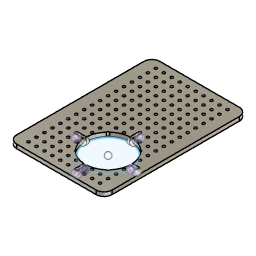
base-plate-2 (Autodesk Fusion 360 design; units mm, degrees)
part number: 2026-04-18-13-53-20-115
Autodesk Fusion 360 part; units mm, degrees
sketch "Sketch1" plane through (0, 0, 0) normal (0, 0, 1) x (1, 0, 0)
  line L0 (10, 0) -> (110, 0)
  line L1 (120, 10) -> (120, 170)
  line L2 (110, 180) -> (10, 180)
  line L3 (0, 170) -> (0, 10)
  arc A0 (10, 180) -> (0, 170) centre (10, 170) ccw
  arc A1 (120, 170) -> (110, 180) centre (110, 170) ccw
  arc A2 (110, 0) -> (120, 10) centre (110, 10) ccw
  arc A3 (0, 10) -> (10, 0) centre (10, 10) ccw
  circle A4 centre (15, 170) radius 1.625
  circle A5 centre (25, 170) radius 1.625
  circle A6 centre (35, 170) radius 1.625
  circle A7 centre (45, 170) radius 1.625
  circle A8 centre (65, 170) radius 1.625
  circle A9 centre (55, 170) radius 1.625
  circle A10 centre (35, 100) radius 1.625
  circle A11 centre (25, 100) radius 1.625
  circle A12 centre (15, 100) radius 1.625
  circle A13 centre (55, 100) radius 1.625
  circle A14 centre (65, 100) radius 1.625
  circle A15 centre (45, 100) radius 1.625
  circle A16 centre (15, 90) radius 1.625
  circle A17 centre (65, 90) radius 1.625
  circle A18 centre (65, 80) radius 1.625
  circle A19 centre (25, 90) radius 1.625
  circle A20 centre (45, 80) radius 1.625
  circle A21 centre (15, 80) radius 1.625
  circle A22 centre (35, 80) radius 1.625
  circle A23 centre (35, 90) radius 1.625
  circle A24 centre (55, 80) radius 1.625
  circle A25 centre (45, 90) radius 1.625
  circle A26 centre (25, 80) radius 1.625
  circle A27 centre (55, 90) radius 1.625
  circle A28 centre (35, 50) radius 1.625
  circle A29 centre (15, 50) radius 1.625
  circle A30 centre (65, 40) radius 1.625
  circle A31 centre (35, 40) radius 1.625
  circle A32 centre (25, 60) radius 1.625
  circle A33 centre (25, 50) radius 1.625
  circle A34 centre (45, 40) radius 1.625
  circle A35 centre (45, 60) radius 1.625
  circle A36 centre (15, 40) radius 1.625
  circle A37 centre (65, 50) radius 1.625
  circle A38 centre (25, 40) radius 1.625
  circle A39 centre (55, 50) radius 1.625
  circle A40 centre (45, 50) radius 1.625
  circle A41 centre (55, 40) radius 1.625
  circle A42 centre (15, 70) radius 1.625
  circle A43 centre (45, 70) radius 1.625
  circle A44 centre (65, 60) radius 1.625
  circle A45 centre (25, 70) radius 1.625
  circle A46 centre (55, 70) radius 1.625
  circle A47 centre (65, 70) radius 1.625
  circle A48 centre (15, 60) radius 1.625
  circle A49 centre (55, 60) radius 1.625
  circle A50 centre (35, 60) radius 1.625
  circle A51 centre (35, 70) radius 1.625
  circle A52 centre (25, 10) radius 1.625
  circle A53 centre (55, 20) radius 1.625
  circle A54 centre (25, 20) radius 1.625
  circle A55 centre (35, 20) radius 1.625
  circle A56 centre (35, 30) radius 1.625
  circle A57 centre (55, 30) radius 1.625
  circle A58 centre (55, 10) radius 1.625
  circle A59 centre (15, 30) radius 1.625
  circle A60 centre (65, 30) radius 1.625
  circle A61 centre (45, 10) radius 1.625
  circle A62 centre (15, 10) radius 1.625
  circle A63 centre (45, 20) radius 1.625
  circle A64 centre (45, 30) radius 1.625
  circle A65 centre (15, 20) radius 1.625
  circle A66 centre (65, 10) radius 1.625
  circle A67 centre (65, 20) radius 1.625
  circle A68 centre (35, 10) radius 1.625
  circle A69 centre (25, 30) radius 1.625
  circle A70 centre (35, 110) radius 1.625
  circle A71 centre (65, 110) radius 1.625
  circle A72 centre (15, 120) radius 1.625
  circle A73 centre (65, 120) radius 1.625
  circle A74 centre (45, 120) radius 1.625
  circle A75 centre (25, 130) radius 1.625
  circle A76 centre (55, 130) radius 1.625
  circle A77 centre (25, 110) radius 1.625
  circle A78 centre (65, 140) radius 1.625
  circle A79 centre (25, 120) radius 1.625
  circle A80 centre (35, 140) radius 1.625
  circle A81 centre (15, 140) radius 1.625
  circle A82 centre (15, 130) radius 1.625
  circle A83 centre (25, 140) radius 1.625
  circle A84 centre (45, 130) radius 1.625
  circle A85 centre (55, 140) radius 1.625
  circle A86 centre (55, 110) radius 1.625
  circle A87 centre (65, 130) radius 1.625
  circle A88 centre (45, 140) radius 1.625
  circle A89 centre (45, 110) radius 1.625
  circle A90 centre (35, 120) radius 1.625
  circle A91 centre (15, 110) radius 1.625
  circle A92 centre (55, 120) radius 1.625
  circle A93 centre (35, 130) radius 1.625
  circle A94 centre (45, 150) radius 1.625
  circle A95 centre (65, 140) radius 1.625
  circle A96 centre (55, 140) radius 1.625
  circle A97 centre (65, 150) radius 1.625
  circle A98 centre (45, 140) radius 1.625
  circle A99 centre (55, 150) radius 1.625
  circle A100 centre (55, 160) radius 1.625
  circle A101 centre (35, 140) radius 1.625
  circle A102 centre (35, 150) radius 1.625
  circle A103 centre (35, 160) radius 1.625
  circle A104 centre (15, 140) radius 1.625
  circle A105 centre (25, 140) radius 1.625
  circle A106 centre (45, 160) radius 1.625
  circle A107 centre (15, 160) radius 1.625
  circle A108 centre (15, 150) radius 1.625
  circle A109 centre (25, 150) radius 1.625
  circle A110 centre (65, 160) radius 1.625
  circle A111 centre (25, 160) radius 1.625
  circle A112 centre (95, 160) radius 1.625
  circle A113 centre (85, 90) radius 1.625
  circle A114 centre (105, 140) radius 1.625
  circle A115 centre (105, 10) radius 1.625
  circle A116 centre (75, 10) radius 1.625
  circle A117 centre (85, 60) radius 1.625
  circle A118 centre (105, 30) radius 1.625
  circle A119 centre (65, 170) radius 1.625
  circle A120 centre (95, 30) radius 1.625
  circle A121 centre (105, 20) radius 1.625
  circle A122 centre (85, 140) radius 1.625
  circle A123 centre (85, 100) radius 1.625
  circle A124 centre (65, 30) radius 1.625
  circle A125 centre (95, 150) radius 1.625
  circle A126 centre (65, 50) radius 1.625
  circle A127 centre (85, 130) radius 1.625
  circle A128 centre (95, 50) radius 1.625
  circle A129 centre (95, 170) radius 1.625
  circle A130 centre (95, 40) radius 1.625
  circle A131 centre (65, 150) radius 1.625
  circle A132 centre (85, 70) radius 1.625
  circle A133 centre (95, 110) radius 1.625
  circle A134 centre (105, 100) radius 1.625
  circle A135 centre (65, 140) radius 1.625
  circle A136 centre (95, 120) radius 1.625
  circle A137 centre (65, 100) radius 1.625
  circle A138 centre (65, 110) radius 1.625
  circle A139 centre (75, 20) radius 1.625
  circle A140 centre (95, 20) radius 1.625
  circle A141 centre (105, 160) radius 1.625
  circle A142 centre (65, 130) radius 1.625
  circle A143 centre (105, 50) radius 1.625
  circle A144 centre (65, 80) radius 1.625
  circle A145 centre (75, 130) radius 1.625
  circle A146 centre (75, 30) radius 1.625
  circle A147 centre (75, 70) radius 1.625
  circle A148 centre (85, 170) radius 1.625
  circle A149 centre (75, 80) radius 1.625
  circle A150 centre (65, 40) radius 1.625
  circle A151 centre (105, 140) radius 1.625
  circle A152 centre (75, 170) radius 1.625
  circle A153 centre (75, 60) radius 1.625
  circle A154 centre (95, 140) radius 1.625
  circle A155 centre (65, 60) radius 1.625
  circle A156 centre (105, 170) radius 1.625
  circle A157 centre (65, 120) radius 1.625
  circle A158 centre (85, 50) radius 1.625
  circle A159 centre (75, 100) radius 1.625
  circle A160 centre (65, 90) radius 1.625
  circle A161 centre (105, 120) radius 1.625
  circle A162 centre (85, 160) radius 1.625
  circle A163 centre (75, 40) radius 1.625
  circle A164 centre (75, 120) radius 1.625
  circle A165 centre (65, 20) radius 1.625
  circle A166 centre (85, 140) radius 1.625
  circle A167 centre (75, 140) radius 1.625
  circle A168 centre (65, 70) radius 1.625
  circle A169 centre (75, 140) radius 1.625
  circle A170 centre (75, 160) radius 1.625
  circle A171 centre (75, 110) radius 1.625
  circle A172 centre (105, 40) radius 1.625
  circle A173 centre (95, 140) radius 1.625
  circle A174 centre (95, 70) radius 1.625
  circle A175 centre (85, 20) radius 1.625
  circle A176 centre (105, 150) radius 1.625
  circle A177 centre (75, 90) radius 1.625
  circle A178 centre (85, 10) radius 1.625
  circle A179 centre (85, 150) radius 1.625
  circle A180 centre (85, 40) radius 1.625
  circle A181 centre (85, 120) radius 1.625
  circle A182 centre (85, 80) radius 1.625
  circle A183 centre (65, 140) radius 1.625
  circle A184 centre (85, 110) radius 1.625
  circle A185 centre (85, 30) radius 1.625
  circle A186 centre (75, 150) radius 1.625
  circle A187 centre (105, 90) radius 1.625
  circle A188 centre (95, 10) radius 1.625
  circle A189 centre (105, 110) radius 1.625
  circle A190 centre (75, 50) radius 1.625
  circle A191 centre (105, 130) radius 1.625
  circle A192 centre (95, 60) radius 1.625
  circle A193 centre (65, 10) radius 1.625
  circle A194 centre (105, 80) radius 1.625
  circle A195 centre (65, 160) radius 1.625
  circle A196 centre (105, 70) radius 1.625
  circle A197 centre (95, 90) radius 1.625
  circle A198 centre (105, 60) radius 1.625
  circle A199 centre (95, 130) radius 1.625
  circle A200 centre (95, 100) radius 1.625
  circle A201 centre (95, 80) radius 1.625
  point P0 (120, 0)
  point P1 (0, 180)
  point P2 (10, 90)
  point P3 (10, 130)
  dimension "d1" = 120
  dimension "d2" = 180
  dimension "d3" = 10
  dimension "d8" = 3.25
  dimension "d10" = 3.25
  dimension "d11" = 3.25
  dimension "d12" = 3.25
  dimension "d13" = 3.25
  dimension "d14" = 3.25
  dimension "d15" = 10
  dimension "d16" = 3.25
  dimension "d17" = 3.25
  dimension "d18" = 3.25
  dimension "d19" = 3.25
  dimension "d20" = 3.25
  dimension "d21" = 3.25
  dimension "d22" = 3.25
  dimension "d23" = 3.25
  dimension "d24" = 3.25
  dimension "d25" = 3.25
  dimension "d26" = 3.25
  dimension "d27" = 3.25
  dimension "d28" = 3.25
  dimension "d29" = 3.25
  dimension "d30" = 3.25
  dimension "d31" = 3.25
  dimension "d32" = 3.25
  dimension "d33" = 3.25
  dimension "d34" = 3.25
  dimension "d35" = 3.25
  dimension "d36" = 3.25
  dimension "d37" = 3.25
  dimension "d38" = 3.25
  dimension "d39" = 3.25
  dimension "d40" = 3.25
  dimension "d41" = 3.25
  dimension "d42" = 3.25
  dimension "d43" = 3.25
  dimension "d44" = 3.25
  dimension "d45" = 3.25
  dimension "d46" = 3.25
  dimension "d47" = 3.25
  dimension "d48" = 3.25
  dimension "d49" = 3.25
  dimension "d50" = 3.25
  dimension "d51" = 3.25
  dimension "d52" = 3.25
  dimension "d53" = 3.25
  dimension "d54" = 3.25
  dimension "d55" = 3.25
  dimension "d56" = 3.25
  dimension "d57" = 3.25
  dimension "d58" = 3.25
  dimension "d59" = 3.25
  dimension "d60" = 3.25
  dimension "d61" = 3.25
  dimension "d62" = 3.25
  dimension "d63" = 3.25
  dimension "d64" = 3.25
  dimension "d65" = 3.25
  dimension "d66" = 3.25
  dimension "d67" = 3.25
  dimension "d68" = 3.25
  dimension "d69" = 3.25
  dimension "d70" = 3.25
  dimension "d71" = 3.25
  dimension "d72" = 3.25
  dimension "d73" = 3.25
  dimension "d74" = 3.25
  dimension "d75" = 3.25
  dimension "d76" = 3.25
  dimension "d77" = 3.25
  dimension "d78" = 3.25
  dimension "d79" = 3.25
  dimension "d80" = 3.25
  dimension "d81" = 3.25
  dimension "d82" = 3.25
  dimension "d83" = 3.25
  dimension "d84" = 3.25
  dimension "d85" = 3.25
  dimension "d86" = 3.25
  dimension "d87" = 3.25
  dimension "d88" = 3.25
  dimension "d89" = 3.25
  dimension "d90" = 3.25
  dimension "d91" = 3.25
  dimension "d92" = 3.25
  dimension "d93" = 3.25
  dimension "d94" = 3.25
  dimension "d95" = 3.25
  dimension "d96" = 3.25
  dimension "d97" = 3.25
  dimension "d98" = 3.25
  dimension "d99" = 3.25
  dimension "d100" = 3.25
  dimension "d101" = 3.25
  dimension "d102" = 3.25
  dimension "d103" = 3.25
  dimension "d104" = 3.25
  dimension "d105" = 3.25
  dimension "d106" = 3.25
  dimension "d107" = 3.25
  dimension "d108" = 3.25
  dimension "d109" = 3.25
  dimension "d110" = 3.25
  dimension "d111" = 3.25
  dimension "d112" = 3.25
  dimension "d113" = 3.25
  dimension "d114" = 3.25
  dimension "d115" = 3.25
  dimension "d116" = 3.25
  dimension "d117" = 3.25
  dimension "d118" = 3.25
  dimension "d119" = 3.25
  dimension "d120" = 3.25
  dimension "d121" = 3.25
  dimension "d122" = 3.25
  dimension "d123" = 3.25
  dimension "d124" = 3.25
  dimension "d125" = 3.25
  dimension "d126" = 3.25
  dimension "d127" = 3.25
  dimension "d128" = 3.25
  dimension "d129" = 3.25
  dimension "d130" = 3.25
  dimension "d131" = 3.25
  dimension "d132" = 3.25
  dimension "d133" = 3.25
  dimension "d134" = 3.25
  dimension "d135" = 3.25
  dimension "d136" = 3.25
  dimension "d137" = 3.25
  dimension "d138" = 3.25
  dimension "d139" = 3.25
  dimension "d140" = 3.25
  dimension "d141" = 3.25
  dimension "d142" = 3.25
  dimension "d143" = 3.25
  dimension "d144" = 3.25
  dimension "d145" = 3.25
  dimension "d146" = 3.25
  dimension "d147" = 3.25
  dimension "d148" = 3.25
  dimension "d149" = 3.25
  dimension "d150" = 3.25
  dimension "d151" = 3.25
  dimension "d152" = 3.25
  dimension "d153" = 3.25
  dimension "d154" = 3.25
  dimension "d155" = 3.25
  dimension "d156" = 3.25
  dimension "d157" = 3.25
  dimension "d158" = 3.25
  dimension "d159" = 3.25
  dimension "d160" = 3.25
  dimension "d161" = 3.25
  dimension "d162" = 3.25
  dimension "d163" = 3.25
  dimension "d164" = 3.25
  dimension "d165" = 3.25
  dimension "d166" = 3.25
  dimension "d167" = 3.25
  dimension "d168" = 3.25
  dimension "d169" = 3.25
  dimension "d170" = 3.25
  dimension "d171" = 3.25
  dimension "d172" = 3.25
  dimension "d173" = 3.25
  dimension "d174" = 3.25
  dimension "d175" = 3.25
  dimension "d176" = 3.25
  dimension "d177" = 3.25
  dimension "d178" = 3.25
  dimension "d179" = 3.25
  dimension "d180" = 3.25
  dimension "d181" = 3.25
  dimension "d182" = 3.25
  dimension "d183" = 3.25
  dimension "d184" = 3.25
  dimension "d185" = 3.25
  dimension "d186" = 3.25
  dimension "d187" = 3.25
  dimension "d188" = 3.25
  dimension "d189" = 3.25
  dimension "d190" = 3.25
  dimension "d191" = 3.25
  dimension "d192" = 3.25
  dimension "d193" = 3.25
  dimension "d194" = 3.25
  dimension "d195" = 3.25
  dimension "d196" = 3.25
  dimension "d197" = 3.25
  dimension "d198" = 3.25
  dimension "d199" = 3.25
  dimension "d200" = 3.25
  dimension "d201" = 3.25
  dimension "d202" = 3.25
  dimension "d203" = 3.25
  dimension "d204" = 3.25
  dimension "d205" = 3.25
  dimension "d206" = 3.25
  dimension "d207" = 3.25
  constraint horizontal L0
  constraint vertical L1
  constraint horizontal L2
  constraint vertical L3
  constraint coincident P1 L2
  constraint coincident P1 L3
  constraint tangent L2 A0
  constraint tangent L3 A0
  constraint tangent L1 A1
  constraint tangent L2 A1
  constraint equal A0 A1
  constraint coincident P0 L0
  constraint coincident P0 L1
  constraint tangent L0 A2
  constraint tangent L1 A2
  constraint equal A0 A2
  constraint coincident origin L0
  constraint coincident origin L3
  constraint tangent L0 A3
  constraint tangent L3 A3
  constraint equal A0 A3
  constraint horizontal A4.centre A5.centre
  constraint horizontal A6.centre A7.centre
  constraint horizontal A9.centre A8.centre
  constraint horizontal A5.centre A6.centre
  constraint horizontal A7.centre A9.centre
  constraint horizontal A12.centre A11.centre
  constraint horizontal A10.centre A15.centre
  constraint horizontal A13.centre A14.centre
  constraint horizontal A11.centre A10.centre
  constraint horizontal A13.centre A15.centre
  constraint horizontal A16.centre A19.centre
  constraint horizontal A23.centre A25.centre
  constraint horizontal A27.centre A17.centre
  constraint horizontal A19.centre A23.centre
  constraint horizontal A27.centre A25.centre
  constraint horizontal A21.centre A26.centre
  constraint horizontal A22.centre A20.centre
  constraint horizontal A18.centre A24.centre
  constraint horizontal A22.centre A26.centre
  constraint horizontal A24.centre A20.centre
  constraint horizontal A42.centre A45.centre
  constraint horizontal A51.centre A43.centre
  constraint horizontal A46.centre A47.centre
  constraint horizontal A45.centre A51.centre
  constraint horizontal A46.centre A43.centre
  constraint horizontal A48.centre A32.centre
  constraint horizontal A50.centre A35.centre
  constraint horizontal A44.centre A49.centre
  constraint horizontal A50.centre A32.centre
  constraint horizontal A49.centre A35.centre
  constraint horizontal A29.centre A33.centre
  constraint horizontal A28.centre A40.centre
  constraint horizontal A37.centre A39.centre
  constraint horizontal A28.centre A33.centre
  constraint horizontal A40.centre A39.centre
  constraint horizontal A36.centre A38.centre
  constraint horizontal A31.centre A34.centre
  constraint horizontal A30.centre A41.centre
  constraint horizontal A38.centre A31.centre
  constraint horizontal A41.centre A34.centre
  constraint horizontal A59.centre A69.centre
  constraint horizontal A56.centre A64.centre
  constraint horizontal A57.centre A60.centre
  constraint horizontal A69.centre A56.centre
  constraint horizontal A57.centre A64.centre
  constraint horizontal A65.centre A54.centre
  constraint horizontal A55.centre A63.centre
  constraint horizontal A67.centre A53.centre
  constraint horizontal A55.centre A54.centre
  constraint horizontal A53.centre A63.centre
  constraint horizontal A62.centre A52.centre
  constraint horizontal A68.centre A61.centre
  constraint horizontal A66.centre A58.centre
  constraint horizontal A68.centre A52.centre
  constraint horizontal A61.centre A58.centre
  constraint horizontal A81.centre A83.centre
  constraint horizontal A80.centre A88.centre
  constraint horizontal A78.centre A85.centre
  constraint horizontal A80.centre A83.centre
  constraint horizontal A85.centre A88.centre
  constraint horizontal A82.centre A75.centre
  constraint horizontal A93.centre A84.centre
  constraint horizontal A87.centre A76.centre
  constraint horizontal A93.centre A75.centre
  constraint horizontal A84.centre A76.centre
  constraint horizontal A72.centre A79.centre
  constraint horizontal A90.centre A74.centre
  constraint horizontal A73.centre A92.centre
  constraint horizontal A79.centre A90.centre
  constraint horizontal A92.centre A74.centre
  constraint horizontal A77.centre A91.centre
  constraint horizontal A89.centre A70.centre
  constraint horizontal A86.centre A71.centre
  constraint horizontal A77.centre A70.centre
  constraint horizontal A86.centre A89.centre
  constraint horizontal A111.centre A107.centre
  constraint horizontal A106.centre A103.centre
  constraint horizontal A100.centre A110.centre
  constraint horizontal A111.centre A103.centre
  constraint horizontal A100.centre A106.centre
  constraint horizontal A108.centre A109.centre
  constraint horizontal A102.centre A94.centre
  constraint horizontal A97.centre A99.centre
  constraint horizontal A102.centre A109.centre
  constraint horizontal A94.centre A99.centre
  constraint horizontal A83.centre A81.centre
  constraint horizontal A83.centre A80.centre
  constraint horizontal A88.centre A85.centre
  constraint horizontal A152.centre A148.centre
  constraint horizontal A129.centre A156.centre
  constraint horizontal A8.centre A152.centre
  constraint horizontal A129.centre A148.centre
  constraint horizontal A159.centre A123.centre
  constraint horizontal A134.centre A200.centre
  constraint horizontal A159.centre A14.centre
  constraint horizontal A200.centre A123.centre
  constraint horizontal A177.centre A113.centre
  constraint horizontal A187.centre A197.centre
  constraint horizontal A177.centre A17.centre
  constraint horizontal A113.centre A197.centre
  constraint horizontal A149.centre A182.centre
  constraint horizontal A194.centre A201.centre
  constraint horizontal A18.centre A149.centre
  constraint horizontal A201.centre A182.centre
  constraint horizontal A132.centre A147.centre
  constraint horizontal A174.centre A196.centre
  constraint horizontal A47.centre A147.centre
  constraint horizontal A174.centre A132.centre
  constraint horizontal A117.centre A153.centre
  constraint horizontal A198.centre A192.centre
  constraint horizontal A44.centre A153.centre
  constraint horizontal A117.centre A192.centre
  constraint horizontal A158.centre A190.centre
  constraint horizontal A143.centre A128.centre
  constraint horizontal A37.centre A190.centre
  constraint horizontal A158.centre A128.centre
  constraint horizontal A163.centre A180.centre
  constraint horizontal A172.centre A130.centre
  constraint horizontal A163.centre A30.centre
  constraint horizontal A130.centre A180.centre
  constraint horizontal A146.centre A185.centre
  constraint horizontal A118.centre A120.centre
  constraint horizontal A60.centre A146.centre
  constraint horizontal A185.centre A120.centre
  constraint horizontal A139.centre A175.centre
  constraint horizontal A121.centre A140.centre
  constraint horizontal A139.centre A67.centre
  constraint horizontal A175.centre A140.centre
  constraint horizontal A116.centre A178.centre
  constraint horizontal A188.centre A115.centre
  constraint horizontal A116.centre A66.centre
  constraint horizontal A188.centre A178.centre
  constraint horizontal A122.centre A167.centre
  constraint horizontal A154.centre A114.centre
  constraint horizontal A78.centre A167.centre
  constraint horizontal A154.centre A122.centre
  constraint horizontal A145.centre A127.centre
  constraint horizontal A191.centre A199.centre
  constraint horizontal A145.centre A87.centre
  constraint horizontal A127.centre A199.centre
  constraint horizontal A164.centre A181.centre
  constraint horizontal A161.centre A136.centre
  constraint horizontal A73.centre A164.centre
  constraint horizontal A181.centre A136.centre
  constraint horizontal A184.centre A171.centre
  constraint horizontal A133.centre A189.centre
  constraint horizontal A171.centre A71.centre
  constraint horizontal A184.centre A133.centre
  constraint horizontal A162.centre A170.centre
  constraint horizontal A141.centre A112.centre
  constraint horizontal A110.centre A170.centre
  constraint horizontal A162.centre A112.centre
  constraint horizontal A186.centre A179.centre
  constraint horizontal A176.centre A125.centre
  constraint horizontal A186.centre A97.centre
  constraint horizontal A179.centre A125.centre
  constraint horizontal A167.centre A122.centre
  constraint horizontal A114.centre A154.centre
  constraint horizontal A122.centre A154.centre
  measures "d1" distance of origin P0
  measures "d2" distance of origin P1
  measures "d3" radius of A0
  measures "d8" diameter of A4
  measures "d10" diameter of A5
  measures "d11" diameter of A6
  measures "d12" diameter of A7 A91.centre
  measures "d13" diameter of A9 A91.centre
  measures "d14" diameter of A8 A91.centre
  measures "d15" distance of L2 A4.centre
  measures "d16" diameter of A12
  measures "d17" diameter of A11
  measures "d18" diameter of A10
  measures "d19" diameter of A15 A91.centre
  measures "d20" diameter of A13 A91.centre
  measures "d21" diameter of A14 A91.centre
  measures "d22" diameter of A16
  measures "d23" diameter of A19
  measures "d24" diameter of A23
  measures "d25" diameter of A25 A91.centre
  measures "d26" diameter of A27 A91.centre
  measures "d27" diameter of A17 A91.centre
  measures "d28" diameter of A21
  measures "d29" diameter of A26
  measures "d30" diameter of A22
  measures "d31" diameter of A20 A91.centre
  measures "d32" diameter of A24 A91.centre
  measures "d33" diameter of A18 A91.centre
  measures "d34" diameter of A42
  measures "d35" diameter of A45
  measures "d36" diameter of A51
  measures "d37" diameter of A43 A91.centre
  measures "d38" diameter of A46 A91.centre
  measures "d39" diameter of A47 A91.centre
  measures "d40" diameter of A48
  measures "d41" diameter of A32
  measures "d42" diameter of A50
  measures "d43" diameter of A35 A91.centre
  measures "d44" diameter of A49 A91.centre
  measures "d45" diameter of A44 A91.centre
  measures "d46" diameter of A29
  measures "d47" diameter of A33
  measures "d48" diameter of A28
  measures "d49" diameter of A40 A91.centre
  measures "d50" diameter of A39 A91.centre
  measures "d51" diameter of A37 A91.centre
  measures "d52" diameter of A36
  measures "d53" diameter of A38
  measures "d54" diameter of A31
  measures "d55" diameter of A34 A91.centre
  measures "d56" diameter of A41 A91.centre
  measures "d57" diameter of A30 A91.centre
  measures "d58" diameter of A59
  measures "d59" diameter of A69
  measures "d60" diameter of A56
  measures "d61" diameter of A64 A91.centre
  measures "d62" diameter of A57 A91.centre
  measures "d63" diameter of A60 A91.centre
  measures "d64" diameter of A65
  measures "d65" diameter of A54
  measures "d66" diameter of A55
  measures "d67" diameter of A63 A91.centre
  measures "d68" diameter of A53 A91.centre
  measures "d69" diameter of A67 A91.centre
  measures "d70" diameter of A62
  measures "d71" diameter of A52
  measures "d72" diameter of A68
  measures "d73" diameter of A61 A91.centre
  measures "d74" diameter of A58 A91.centre
  measures "d75" diameter of A66 A91.centre
  measures "d76" diameter of A81
  measures "d77" diameter of A83
  measures "d78" diameter of A80
  measures "d79" diameter of A88 A91.centre
  measures "d80" diameter of A85 A91.centre
  measures "d81" diameter of A78 A91.centre
  measures "d82" diameter of A82
  measures "d83" diameter of A75
  measures "d84" diameter of A93
  measures "d85" diameter of A84 A91.centre
  measures "d86" diameter of A76 A91.centre
  measures "d87" diameter of A87 A91.centre
  measures "d88" diameter of A72
  measures "d89" diameter of A79
  measures "d90" diameter of A90
  measures "d91" diameter of A74 A91.centre
  measures "d92" diameter of A92 A91.centre
  measures "d93" diameter of A73 A91.centre
  measures "d94" diameter of A91
  measures "d95" diameter of A77
  measures "d96" diameter of A70
  measures "d97" diameter of A89 A91.centre
  measures "d98" diameter of A86 A91.centre
  measures "d99" diameter of A71 A91.centre
  measures "d100" diameter of A107
  measures "d101" diameter of A111
  measures "d102" diameter of A103
  measures "d103" diameter of A106 A91.centre
  measures "d104" diameter of A100 A91.centre
  measures "d105" diameter of A110 A91.centre
  measures "d106" diameter of A108
  measures "d107" diameter of A109
  measures "d108" diameter of A102
  measures "d109" diameter of A94 A91.centre
  measures "d110" diameter of A99 A91.centre
  measures "d111" diameter of A97 A91.centre
  measures "d112" diameter of A104
  measures "d113" diameter of A105
  measures "d114" diameter of A101
  measures "d115" diameter of A98 A91.centre
  measures "d116" diameter of A96 A91.centre
  measures "d117" diameter of A95 A91.centre
  measures "d108" diameter of A119
  measures "d108" diameter of A152
  measures "d120" diameter of A148
  measures "d121" diameter of A129
  measures "d122" diameter of A156
  measures "d108" diameter of A137
  measures "d108" diameter of A159
  measures "d125" diameter of A123
  measures "d126" diameter of A200
  measures "d127" diameter of A134
  measures "d108" diameter of A160
  measures "d108" diameter of A177
  measures "d130" diameter of A113
  measures "d131" diameter of A197
  measures "d132" diameter of A187
  measures "d108" diameter of A144
  measures "d108" diameter of A149
  measures "d135" diameter of A182
  measures "d136" diameter of A201
  measures "d137" diameter of A194
  measures "d108" diameter of A168
  measures "d108" diameter of A147
  measures "d140" diameter of A132
  measures "d141" diameter of A174
  measures "d142" diameter of A196
  measures "d108" diameter of A155
  measures "d108" diameter of A153
  measures "d145" diameter of A117
  measures "d146" diameter of A192
  measures "d147" diameter of A198
  measures "d108" diameter of A126
  measures "d108" diameter of A190
  measures "d150" diameter of A158
  measures "d151" diameter of A128
  measures "d152" diameter of A143
  measures "d108" diameter of A150
  measures "d108" diameter of A163
  measures "d155" diameter of A180
  measures "d156" diameter of A130
  measures "d157" diameter of A172
  measures "d108" diameter of A124
  measures "d108" diameter of A146
  measures "d160" diameter of A185
  measures "d161" diameter of A120
  measures "d162" diameter of A118
  measures "d108" diameter of A165
  measures "d108" diameter of A139
  measures "d165" diameter of A175
  measures "d166" diameter of A140
  measures "d167" diameter of A121
  measures "d108" diameter of A193
  measures "d108" diameter of A116
  measures "d170" diameter of A178
  measures "d171" diameter of A188
  measures "d172" diameter of A115
  measures "d108" diameter of A135
  measures "d108" diameter of A167
  measures "d175" diameter of A166
  measures "d176" diameter of A154
  measures "d177" diameter of A151
  measures "d108" diameter of A142
  measures "d108" diameter of A145
  measures "d180" diameter of A127
  measures "d181" diameter of A199
  measures "d182" diameter of A191
  measures "d108" diameter of A157
  measures "d108" diameter of A164
  measures "d185" diameter of A181
  measures "d186" diameter of A136
  measures "d187" diameter of A161
  measures "d108" diameter of A138
  measures "d108" diameter of A171
  measures "d190" diameter of A184
  measures "d191" diameter of A133
  measures "d192" diameter of A189
  measures "d108" diameter of A195
  measures "d108" diameter of A170
  measures "d195" diameter of A162
  measures "d196" diameter of A112
  measures "d197" diameter of A141
  measures "d108" diameter of A131
  measures "d108" diameter of A186
  measures "d200" diameter of A179
  measures "d201" diameter of A125
  measures "d202" diameter of A176
  measures "d108" diameter of A183
  measures "d108" diameter of A169
  measures "d205" diameter of A122
  measures "d206" diameter of A173
  measures "d207" diameter of A114
sketch "Sketch2" plane through (0, 0, 0) normal (0, 0, 1) x (1, 0, 0)
  circle A0 centre (75, 50) radius 28
  line L0 (73.375, 10) -> (73.375, 20)
  circle A1 centre (75, 20) radius 1.625
  line L1 (76.625, 10.0087) -> (76.625, 20)
  circle A2 centre (75, 10) radius 1.625
  line L2 (35, 51.625) -> (45, 51.625)
  line L3 (35, 48.375) -> (45, 48.375)
  circle A3 centre (35, 50) radius 1.625
  line L4 (73.375, 90) -> (73.375, 80)
  line L5 (76.625, 90) -> (76.625, 80)
  circle A4 centre (75, 90) radius 1.625
  circle A5 centre (112, 50) radius 1.625
  line L6 (105, 51.625) -> (112, 51.625)
  line L7 (105, 48.375) -> (112, 48.375)
  circle A6 centre (105, 50) radius 1.625
  point P0 (105, 50)
  dimension "d208" = 56
  dimension "d209" = 3.25
  dimension "d210" = 7
  constraint vertical L0
  constraint tangent L0 A1
  constraint coincident A1 L1.end
  constraint tangent A1 L1
  constraint tangent L1 A2
  constraint horizontal L2
  constraint horizontal L3
  constraint tangent L2 A3
  constraint tangent L3 A3
  constraint vertical L4
  constraint parallel L4 L5
  constraint tangent L4 A4
  constraint tangent L5 A4
  constraint horizontal L6
  constraint parallel L6 L7
  constraint tangent L6 A6
  constraint tangent L7 A6
  measures "d208" diameter of A0
  measures "d209" diameter of A5
  measures "d210" distance of A5.centre P0
extrude "Extrude1" add sketch "Sketch1" along normal blind 5
sketch "Sketch3" plane through (0, 0, 5) normal (0, 0, 1) x (-1, 0, 0)
  circle A0 centre (-105, -70) radius 1.625
  circle A1 centre (-35, -20) radius 1.625
  circle A2 centre (-95, -70) radius 1.625
  circle A3 centre (-85, -120) radius 1.625
  circle A4 centre (-65, -100) radius 1.625
  circle A5 centre (-105, -150) radius 1.625
  circle A6 centre (-45, -150) radius 1.625
  circle A7 centre (-25, -60) radius 1.625
  circle A8 centre (-85, -110) radius 1.625
  circle A9 centre (-45, -20) radius 1.625
  circle A10 centre (-65, -90) radius 1.625
  circle A11 centre (-65, -110) radius 1.625
  circle A12 centre (-45, -120) radius 1.625
  circle A13 centre (-65, -60) radius 1.625
  circle A14 centre (-65, -120) radius 1.625
  circle A15 centre (-85, -50) radius 1.625
  circle A16 centre (-75, -100) radius 1.625
  circle A17 centre (-35, -100) radius 1.625
  circle A18 centre (-105, -170) radius 1.625
  circle A19 centre (-75, -20) radius 1.625
  circle A20 centre (-95, -120) radius 1.625
  circle A21 centre (-55, -100) radius 1.625
  circle A22 centre (-15, -20) radius 1.625
  circle A23 centre (-15, -100) radius 1.625
  circle A24 centre (-15, -50) radius 1.625
  circle A25 centre (-45, -170) radius 1.625
  circle A26 centre (-105, -120) radius 1.625
  circle A27 centre (-95, -10) radius 1.625
  circle A28 centre (-75, -90) radius 1.625
  circle A29 centre (-95, -60) radius 1.625
  circle A30 centre (-55, -80) radius 1.625
  circle A31 centre (-15, -10) radius 1.625
  circle A32 centre (-25, -170) radius 1.625
  circle A33 centre (-45, -130) radius 1.625
  circle A34 centre (-65, -20) radius 1.625
  circle A35 centre (-75, -10) radius 1.625
  circle A36 centre (-75, -40) radius 1.625
  circle A37 centre (-85, -10) radius 1.625
  circle A38 centre (-25, -100) radius 1.625
  circle A39 centre (-25, -130) radius 1.625
  circle A40 centre (-55, -170) radius 1.625
  circle A41 centre (-75, -130) radius 1.625
  circle A42 centre (-105, -40) radius 1.625
  circle A43 centre (-35, -170) radius 1.625
  circle A44 centre (-95, -80) radius 1.625
  circle A45 centre (-85, -20) radius 1.625
  circle A46 centre (-25, -150) radius 1.625
  circle A47 centre (-75, -70) radius 1.625
  circle A48 centre (-85, -160) radius 1.625
  circle A49 centre (-25, -30) radius 1.625
  circle A50 centre (-75, -160) radius 1.625
  circle A51 centre (-65, -40) radius 1.625
  circle A52 centre (-15, -170) radius 1.625
  circle A53 centre (-25, -120) radius 1.625
  circle A54 centre (-95, -100) radius 1.625
  circle A55 centre (-15, -110) radius 1.625
  circle A56 centre (-75, -150) radius 1.625
  circle A57 centre (-105, -60) radius 1.625
  circle A58 centre (-15, -130) radius 1.625
  circle A59 centre (-105, -130) radius 1.625
  circle A60 centre (-35, -110) radius 1.625
  circle A61 centre (-45, -110) radius 1.625
  circle A62 centre (-35, -40) radius 1.625
  circle A63 centre (-75, -50) radius 1.625
  circle A64 centre (-15, -120) radius 1.625
  circle A65 centre (-95, -160) radius 1.625
  circle A66 centre (-35, -150) radius 1.625
  circle A67 centre (-35, -140) radius 1.625
  circle A68 centre (-55, -120) radius 1.625
  circle A69 centre (-105, -80) radius 1.625
  circle A70 centre (-75, -120) radius 1.625
  circle A71 centre (-45, -80) radius 1.625
  circle A72 centre (-95, -90) radius 1.625
  circle A73 centre (-85, -140) radius 1.625
  circle A74 centre (-105, -140) radius 1.625
  circle A75 centre (-85, -30) radius 1.625
  circle A76 centre (-75, -30) radius 1.625
  circle A77 centre (-45, -40) radius 1.625
  circle A78 centre (-35, -70) radius 1.625
  circle A79 centre (-105, -30) radius 1.625
  circle A80 centre (-55, -150) radius 1.625
  circle A81 centre (-85, -80) radius 1.625
  circle A82 centre (-95, -110) radius 1.625
  circle A83 centre (-65, -130) radius 1.625
  circle A84 centre (-25, -50) radius 1.625
  circle A85 centre (-105, -100) radius 1.625
  circle A86 centre (-25, -110) radius 1.625
  circle A87 centre (-25, -20) radius 1.625
  circle A88 centre (-105, -10) radius 1.625
  circle A89 centre (-55, -20) radius 1.625
  circle A90 centre (-25, -80) radius 1.625
  circle A91 centre (-95, -20) radius 1.625
  circle A92 centre (-25, -10) radius 1.625
  circle A93 centre (-85, -90) radius 1.625
  circle A94 centre (-35, -50) radius 1.625
  circle A95 centre (-65, -80) radius 1.625
  circle A96 centre (-25, -160) radius 1.625
  circle A97 centre (-55, -90) radius 1.625
  circle A98 centre (-105, -110) radius 1.625
  circle A99 centre (-55, -160) radius 1.625
  circle A100 centre (-85, -40) radius 1.625
  circle A101 centre (-105, -50) radius 1.625
  circle A102 centre (-75, -110) radius 1.625
  circle A103 centre (-55, -140) radius 1.625
  circle A104 centre (-65, -160) radius 1.625
  circle A105 centre (-15, -80) radius 1.625
  circle A106 centre (-35, -10) radius 1.625
  circle A107 centre (-35, -120) radius 1.625
  circle A108 centre (-85, -70) radius 1.625
  circle A109 centre (-45, -60) radius 1.625
  circle A110 centre (-65, -170) radius 1.625
  circle A111 centre (-75, -140) radius 1.625
  circle A112 centre (-65, -150) radius 1.625
  circle A113 centre (-15, -40) radius 1.625
  circle A114 centre (-55, -130) radius 1.625
  circle A115 centre (-95, -40) radius 1.625
  circle A116 centre (-45, -30) radius 1.625
  circle A117 centre (-25, -40) radius 1.625
  circle A118 centre (-45, -90) radius 1.625
  circle A119 centre (-55, -110) radius 1.625
  circle A120 centre (-95, -170) radius 1.625
  circle A121 centre (-85, -60) radius 1.625
  circle A122 centre (-65, -10) radius 1.625
  circle A123 centre (-55, -50) radius 1.625
  circle A124 centre (-45, -70) radius 1.625
  circle A125 centre (-95, -30) radius 1.625
  circle A126 centre (-15, -30) radius 1.625
  circle A127 centre (-35, -60) radius 1.625
  circle A128 centre (-45, -160) radius 1.625
  circle A129 centre (-35, -130) radius 1.625
  circle A130 centre (-55, -10) radius 1.625
  circle A131 centre (-55, -30) radius 1.625
  circle A132 centre (-15, -60) radius 1.625
  circle A133 centre (-15, -150) radius 1.625
  circle A134 centre (-15, -140) radius 1.625
  circle A135 centre (-45, -10) radius 1.625
  circle A136 centre (-105, -20) radius 1.625
  circle A137 centre (-105, -160) radius 1.625
  circle A138 centre (-25, -140) radius 1.625
  circle A139 centre (-85, -100) radius 1.625
  circle A140 centre (-55, -60) radius 1.625
  circle A141 centre (-95, -130) radius 1.625
  circle A142 centre (-65, -30) radius 1.625
  circle A143 centre (-75, -60) radius 1.625
  circle A144 centre (-45, -100) radius 1.625
  circle A145 centre (-75, -170) radius 1.625
  circle A146 centre (-45, -140) radius 1.625
  circle A147 centre (-85, -130) radius 1.625
  circle A148 centre (-65, -140) radius 1.625
  circle A149 centre (-95, -50) radius 1.625
  circle A150 centre (-35, -30) radius 1.625
  circle A151 centre (-45, -50) radius 1.625
  circle A152 centre (-65, -70) radius 1.625
  circle A153 centre (-15, -160) radius 1.625
  circle A154 centre (-55, -40) radius 1.625
  circle A155 centre (-75, -80) radius 1.625
  circle A156 centre (-65, -50) radius 1.625
  circle A157 centre (-95, -140) radius 1.625
  circle A158 centre (-15, -70) radius 1.625
  circle A159 centre (-105, -90) radius 1.625
  circle A160 centre (-15, -90) radius 1.625
  circle A161 centre (-25, -90) radius 1.625
  circle A162 centre (-95, -150) radius 1.625
  circle A163 centre (-85, -150) radius 1.625
  circle A164 centre (-35, -160) radius 1.625
  circle A165 centre (-55, -70) radius 1.625
  circle A166 centre (-25, -70) radius 1.625
  circle A167 centre (-85, -170) radius 1.625
  circle A168 centre (-35, -80) radius 1.625
  circle A169 centre (-35, -90) radius 1.625
  arc A170 (0, -10) -> (-10, 0) centre (-10, -10) ccw
  line L0 (-10, 0) -> (-110, 0)
  arc A171 (-110, 0) -> (-120, -10) centre (-110, -10) ccw
  line L1 (-120, -10) -> (-120, -170)
  arc A172 (-120, -170) -> (-110, -180) centre (-110, -170) ccw
  line L2 (-110, -180) -> (-10, -180)
  arc A173 (-10, -180) -> (0, -170) centre (-10, -170) ccw
  line L3 (0, -170) -> (0, -10)
  circle A174 centre (-75, -50) radius 29
  line L4 (-73.375, -90) -> (-73.375, -80)
  line L5 (-76.625, -90) -> (-76.625, -80)
  line L6 (-35.0185, -51.6249) -> (-45, -51.625)
  line L7 (-35.0185, -48.3751) -> (-45, -48.375)
  circle A175 centre (-112.2545, -50) radius 1.625
  line L8 (-105.0194, -51.6249) -> (-112, -51.6249)
  line L9 (-105.0193, -48.3751) -> (-112.2545, -48.375)
  line L10 (-73.4014, -19.7082) -> (-73.375, -10.0044)
  line L11 (-76.5986, -19.7082) -> (-76.625, -10.0044)
  line L12 (-105.0194, -51.6249) -> (-112, -51.6249)
  line L13 (-105.0193, -48.3751) -> (-112.2545, -48.375)
  dimension "d213" = 58
  dimension "d214" = 3.25
  constraint concentric A63 A174
  constraint coincident A28 L4.start
  constraint coincident A155 L4.end
  constraint tangent A155 L4
  constraint vertical L4
  constraint coincident A28 L5.start
  constraint coincident A155 L5.end
  constraint tangent A155 L5
  constraint parallel L4 L5
  constraint coincident A94 L6.start
  constraint coincident A151 L6.end
  constraint tangent A151 L6
  constraint coincident A94 L7.start
  constraint coincident A151 L7.end
  constraint tangent A151 L7
  constraint coincident A101 L8.start
  constraint horizontal L8
  constraint coincident A101 L9.start
  constraint coincident A175 L9.end
  constraint tangent A175 L9
  constraint coincident A19 L10.start
  constraint coincident A35 L10.end
  constraint tangent A35 L10
  constraint coincident A19 L11.start
  constraint coincident A35 L11.end
  constraint tangent A35 L11
  measures "d214" diameter of A175
sketch "Sketch4" plane through (0, 0, 5) normal (0, 0, 1) x (-1, 0, 0)
  line L0 (-105, -51.625) -> (-112.2319, -51.625)
  line L1 (-112.2319, -51.625) -> (-112.2319, -48.375)
  line L2 (-112.2319, -48.375) -> (-105, -48.375)
  line L3 (-105, -48.375) -> (-105, -51.625)
  circle A0 centre (-105, -50) radius 1.625
  constraint horizontal L0
  constraint vertical L1
  constraint horizontal L2
  constraint vertical L3
  constraint tangent L0 A0
  constraint tangent L2 A0
extrude "Extrude2" cut sketch "Sketch4" sketch "Sketch3" against normal blind 6 contours L0 L1 L2 A0 of sketch 2 contours A2 A19 A101 A125 A131 A151 A155 A165 A174 | A28 A155 L4 L5 | A19 A35 L10 L11 | A94 A151 L6 L7 | A175
